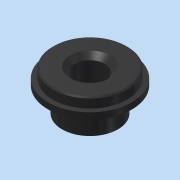
# Autodesk Inventor part: lens
Saved by Autodesk Inventor 2014 (Build 180170000, 170)
## iProperties
Created: 2014-02-26
Part Number: lens
Document SubType Name: Modeling
Designer: Robert Davis
Density: 1 g/cm^3
Material: Generic
Appearance: Dark Gray
Author: Robert Davis
Autodesk Inventor part; units mm, degrees
ref_plane "YZ Plane" through (0, 0, 0) normal (1, 0, 0) x (0, 1, 0)
ref_plane "XZ Plane" through (0, 0, 0) normal (0, 1, 0) x (-1, 0, 0)
ref_plane "XY Plane" through (0, 0, 0) normal (0, 0, 1) x (1, 0, 0)
sketch "Sketch1" plane through (0, 0, 0) normal (0, 0, 1) x (1, 0, 0)
  circle A0 centre (0, 0) radius 6.75
  dimension "d0" = 13.5
  constraints: 1 centre point
  measures "d0" diameter of A0
extrude "Extrusion1" add sketch "Sketch1" along normal blind 1
sketch "Sketch2" plane through (0, 0, 1) normal (0, 0, 1) x (1, 0, 0)
  circle A0 centre (0, 0) radius 6.75 projected
  line L0 (-6.75, 6.75) -> (6.75, 6.75) construction
  line L1 (6.75, 6.75) -> (6.75, -6.75) construction
  line L2 (6.75, -6.75) -> (-6.75, -6.75) construction
  line L3 (-6.75, -6.75) -> (-6.75, 6.75) construction
  line L4 (-6.75, 6.75) -> (6.75, -6.75) construction
  dimension "d4" = 13.5
  constraints: 2 coincident, 2 end point, 1 midpoint, 2 other
  measures "d4" distance of L2.end L0.start
decal "Decal1"
sketch "Sketch3" plane through (0, 0, 0) normal (0, 0, -1) x (-1, 0, 0)
  circle A0 centre (0, 0) radius 6
  dimension "d6" = 12
  constraints: 1 centre point
  measures "d6" diameter of A0
extrude "Extrusion2" add sketch "Sketch3" against normal blind 2.6
hole "Hole1" at (0, 0, 2.6) direction (0, 0, -1) diameter 4.8 end through all
chamfer "Chamfer1" distance 0.8 angle 45 1 edges at (0, 2.4, 2.6)
chamfer "Chamfer2" distance 0.2 angle 45 1 edges at (6, 0, 2.6)
sketch "Sketch4" plane through (0, 0, 0) normal (0, 0, -1) x (-1, 0, 0)
  circle A0 centre (0, 0) radius 2.4 projected
  circle A1 centre (0, 0) radius 4.5
  circle A2 centre (0, 0) radius 2.4
  dimension "d24" = 9
  constraints: 2 centre point
  measures "d24" diameter of A1
extrude "Extrusion3" add sketch "Sketch4" along normal blind 3.9
body "Solid1"
